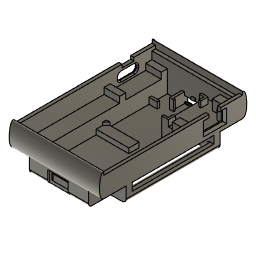
case 9.0 v5 (Autodesk Fusion 360 design; units mm, degrees)
Autodesk Fusion 360 part; units mm, degrees
note: some values were not read from the file. Set by a fixed rule: which face or edge a step refers to.
sketch "case bottom" plane through (0, 0, 0) normal (0, 0, 1) x (1, 0, 0) in component "case"
  line L0 (0, 0) -> (25.8, 0)
  line L1 (25.8, 0) -> (25.8, 34.5)
  line L2 (25.8, 34.5) -> (0, 34.5)
  line L3 (0, 34.5) -> (0, 0)
  line L4 (12.9, 0) -> (12.9, 61.75) construction
  line L5 (8.5, 59.25) -> (17.3, 59.25)
  line L6 (17.3, 59.25) -> (17.3, 64.25)
  line L7 (17.3, 64.25) -> (8.5, 64.25)
  line L8 (8.5, 64.25) -> (8.5, 59.25)
  line L9 (8.5, 59.25) -> (17.3, 64.25) construction
  line L10 (17.3, 59.25) -> (8.5, 64.25) construction
  line L11 (8.35, 64.4) -> (8.35, 59.1)
  line L12 (8.35, 59.1) -> (17.45, 59.1)
  line L13 (17.45, 59.1) -> (17.45, 64.4)
  line L14 (17.45, 64.4) -> (8.35, 64.4)
  line L15 (27.4, 66) -> (-1.6, 66)
  line L16 (-1.6, 66) -> (-1.6, -1.6)
  line L17 (-1.6, -1.6) -> (27.4, -1.6)
  line L18 (27.4, -1.6) -> (27.4, 66)
  line L19 (27.4, 66) -> (-1.6, -1.6) construction
  line L20 (-1.6, 66) -> (27.4, -1.6) construction
  line L21 (-1.6, 32.2) -> (-9.2, 32.2) construction
  line L22 (-9.2, 32.2) -> (-9.2, 12.2)
  line L23 (-5.4, 32.2) -> (-5.4, 12.2)
  line L24 (-5.4, 12.2) -> (-1.6, 12.2)
  line L25 (-1.6, 9.2) -> (-9.2, 9.2)
  line L26 (-9.2, 9.2) -> (-9.2, 12.2)
  line L27 (-5.4, 52.2) -> (-1.6, 52.2)
  line L28 (-5.4, 32.2) -> (-5.4, 52.2)
  line L29 (-1.6, 55.2) -> (-9.2, 55.2)
  line L30 (-9.2, 55.2) -> (-9.2, 52.2)
  line L31 (-9.2, 32.2) -> (-9.2, 52.2)
  line L32 (27.4, 55.2) -> (35, 55.2)
  line L33 (31.2, 52.2) -> (27.4, 52.2)
  line L34 (31.2, 32.2) -> (31.2, 52.2)
  line L35 (35, 55.2) -> (35, 52.2)
  line L36 (35, 32.2) -> (35, 52.2)
  line L37 (31.2, 32.2) -> (31.2, 12.2)
  line L38 (35, 32.2) -> (35, 12.2)
  line L39 (35, 9.2) -> (35, 12.2)
  line L40 (27.4, 9.2) -> (35, 9.2)
  line L41 (31.2, 12.2) -> (27.4, 12.2)
  line L42 (8.35, 64.4) -> (0, 64.4)
  line L43 (0, 64.4) -> (0, 34.5)
  line L44 (17.45, 64.4) -> (25.8, 64.4)
  line L45 (25.8, 64.4) -> (25.8, 34.5)
  line L46 (9.15, 58.3) -> (7.15, 58.3)
  line L47 (7.15, 58.3) -> (7.15, 64.4)
  line L48 (18.65, 58.3) -> (18.65, 64.4)
  line L49 (16.65, 58.3) -> (18.65, 58.3)
  line L50 (25.8, 29.5) -> (0, 29.5)
  line L51 (9.15, 58.3) -> (9.15, 59.1)
  line L52 (16.65, 58.3) -> (16.65, 59.1)
  line L53 (0, 34.5) -> (16, 34.5)
  line L54 (16, 34.5) -> (16, 55.4)
  line L55 (16, 55.4) -> (0, 55.4)
  line L56 (0, 55.4) -> (0, 34.5)
  line L57 (4, 55.4) -> (4, 56.6)
  line L58 (4, 56.6) -> (0, 56.6)
  line L59 (0, 32.7) -> (1.8, 34.5)
  line L60 (0, 32.7) -> (3.5846, 32.7) construction
  line L61 (25.8, 32.7) -> (24, 34.5)
  line L62 (16, 34.5) -> (16, 29.5)
  point P0 (12.9, 43.5)
  point P1 (12.9, 61.75)
  point P2 (12.9, 32.2)
  dimension "d1" = 25.8
  dimension "d2" = 34.5
  dimension "d6" = 8.8
  dimension "d7" = 5
  dimension "d8" = 0.15
  dimension "d10" = 1.6
  dimension "d11" = 1.6
  dimension "d12" = 1.6
  dimension "d13" = 7.6
  dimension "d15" = 3.8
  dimension "d16" = 3
  dimension "d17" = 20
  dimension "d21" = 6.1
  dimension "d23" = 1.2
  dimension "d24" = 5
  dimension "d104" = 29.9
  dimension "d105" = 0.8
  dimension "d106" = 0.8
  dimension "d107" = 16
  dimension "d108" = 20.9
  dimension "d109" = 1.2
  dimension "d110" = 4
  dimension "d155" = 45
  dimension "d156" = 1.8
  constraint horizontal L0
  constraint vertical L1
  constraint horizontal L2
  constraint vertical L3
  constraint coincident L0.start L3.end
  constraint midpoint L0 L4.start
  constraint perpendicular L0 L4
  constraint coincident L4 P0
  constraint horizontal L5
  constraint perpendicular L5 L6
  constraint parallel L5 L7
  constraint parallel L6 L8
  constraint coincident L9 P1
  constraint coincident L10 P1
  constraint coincident P1 L4.end
  constraint horizontal L15
  constraint perpendicular L15 L16
  constraint parallel L15 L17
  constraint parallel L16 L18
  constraint coincident L19 P2
  constraint coincident L20 P2
  constraint coincident L4 P2
  constraint midpoint L16 L21.start
  constraint perpendicular L16 L21
  constraint perpendicular L21 L22
  constraint coincident L21 L23.start
  constraint perpendicular L21 L23
  constraint coincident L16 L24.end
  constraint perpendicular L16 L24
  constraint coincident L16 L25.start
  constraint perpendicular L16 L25
  constraint perpendicular L25 L26
  constraint symmetric L22.start L21 L31.start
  constraint symmetric L21 L22.end L30.end
  constraint symmetric L21 L23.start L28.start
  constraint symmetric L21 L23.end L27.start
  constraint symmetric L21 L24.end L27.end
  constraint symmetric L21 L25.start L29.start
  constraint symmetric L21 L25.end L29.end
  constraint symmetric L4 L21.end L36.start
  constraint symmetric L4 L22.end L38.end
  constraint symmetric L4 L23.start L34.start
  constraint symmetric L4 L23.end L37.end
  constraint symmetric L4 L24.end L41.end
  constraint symmetric L4 L25.start L40.start
  constraint symmetric L4 L25.end L39.start
  constraint symmetric L4 L27.start L33.start
  constraint symmetric L4 L27.end L33.end
  constraint symmetric L4 L29.start L32.start
  constraint symmetric L4 L29.end L32.end
  constraint symmetric L4 L30.end L35.end
  constraint perpendicular L3 L42
  constraint perpendicular L2 L43
  constraint perpendicular L18 L44
  constraint perpendicular L44 L45
  constraint coincident L42 L47.end
  constraint perpendicular L42 L47
  constraint symmetric L4 L46.start L49.start
  constraint symmetric L4 L46.end L48.start
  constraint symmetric L4 L47.end L48.end
  constraint coincident L1 L50.start
  constraint coincident L3 L50.end
  constraint perpendicular L3 L50
  constraint coincident L12 L51.end
  constraint perpendicular L12 L51
  constraint symmetric L4 L51.end L52.end
  constraint horizontal L53
  constraint vertical L54
  constraint horizontal L55
  constraint vertical L56
  constraint coincident L55 L57.start
  constraint perpendicular L55 L57
  constraint coincident L43 L58.end
  constraint perpendicular L43 L58
  constraint horizontal L60
  constraint coincident L3 L59.start
  constraint coincident L53 L59.end
  constraint symmetric L4 L59.start L61.start
  constraint symmetric L4 L59.end L61.end
  constraint coincident L50 L62.end
  constraint perpendicular L50 L62
  measures "d1" distance of L0.start L0.end
  measures "d2" distance of L0.start L2.end
  measures "d6" distance of L6.end L7.end
  measures "d7" distance of L5.start L7.end
  measures "d10" distance of L3 L16
  measures "d11" distance of L0 L17
  measures "d12" distance of L14 L15
  measures "d13" distance of L21.start L21.end
  measures "d15" distance of L16 L23
  measures "d16" distance of L24 L25
  measures "d17" distance of L21 L24
  measures "d21" distance of L46.end L47.end
  measures "d23" distance of L11 L47
  measures "d24" distance of L2 L50
  measures "d104" distance of L2 L42
  measures "d105" distance of L11 L51
  measures "d106" distance of L46.start L51.end
  measures "d107" distance of L2.end L53.end
  measures "d108" distance of L2.end L55.end
  measures "d109" distance of L57.start L57.end
  measures "d110" distance of L57.end L58.end
  measures "d155" angle of L59 L60
  measures "d156" distance of L53 L59.start
extrude "Extrude1" add sketch "case bottom" against normal blind 1.6 contours L0 L1 L3 L50 | L2 L3 L50 L53 L59 L62 | L1 L2 L50 L61 L62 | L2 L3 L53 L59 | L1 L2 L61 | L2 L43 L53 L54 L55 L56 | L2 L12 L42 L43 L44 L45 L46 L47 L48 L49 L51 L52 L54 L55 L57 L58 | L43 L55 L57 L58 | L12 L13 L44 L48 L49 L52 | L11 L12 L13 L14 | L11 L12 L42 L46 L47 L51 | L5 L6 L7 L8 | L15 L16 L17 L18 | L18 L32 L33 L34 L35 L36 L37 L38 L39 L40 L41 | L16 L22 L23 L24 L25 L26 L27 L28 L29 L30 L31 | L18 L33 L34 L37 L41 | L16 L23 L24 L27 L28 makes body 1 in component "case"
extrude "Extrude1'" add sketch "case bottom" along normal blind 3 contours L43 L55 L57 L58 bodies 1 in component "case"
extrude "Extrude2" add sketch "case bottom" along normal blind 5 contours L12 L13 L44 L48 L49 L52 | L11 L12 L42 L46 L47 L51 bodies 1 in component "case"
extrude "Extrude4" add sketch "case bottom" along normal blind 7.6 contours L15 L16 L17 L18 | L18 L32 L33 L34 L35 L36 L37 L38 L39 L40 L41 | L16 L22 L23 L24 L25 L26 L27 L28 L29 L30 L31 | L18 L33 L34 L37 L41 | L16 L23 L24 L27 L28 bodies 1 in component "case"
extrude "Extrude3" add sketch "case bottom" along normal blind 2.4 contours L2 L3 L50 L53 L59 L62 | L2 L3 L53 L59 bodies 1 in component "case"
extrude "Extrude21" add sketch "case bottom" along normal blind 1.4 from surface at 2.4 contours L2 L3 L53 L59 bodies 1 in component "case"
sketch "case top" plane through (0, 0, 7.6) normal (0, 0, 1) x (-1, 0, 0) in component "case"
  line L0 (0, -64.4) -> (-25.8, -64.4)
  line L1 (-25.8, -64.4) -> (-25.8, 0)
  line L2 (-25.8, 0) -> (0, 0)
  line L3 (0, 0) -> (0, -64.4)
  line L4 (1.6, -9.2) -> (1.6, 1.6)
  line L5 (1.6, 1.6) -> (-27.4, 1.6)
  line L6 (-27.4, 1.6) -> (-27.4, -9.2)
  line L7 (-27.4, -9.2) -> (-35, -9.2)
  line L8 (-35, -9.2) -> (-35, -55.2)
  line L9 (-35, -55.2) -> (-27.4, -55.2)
  line L10 (-27.4, -55.2) -> (-27.4, -66)
  line L11 (-27.4, -66) -> (1.6, -66)
  line L12 (1.6, -66) -> (1.6, -55.2)
  line L13 (1.6, -55.2) -> (9.2, -55.2)
  line L14 (9.2, -55.2) -> (9.2, -9.2)
  line L15 (9.2, -9.2) -> (1.6, -9.2)
  line L16 (-12.9, 0) -> (-12.9, -61.75) construction
  line L17 (-25.8, 0) -> (0, 0)
  line L18 (7.6, 0) -> (-33.4, 0)
  line L19 (-33.4, 0) -> (-33.4, -41)
  line L20 (-33.4, -41) -> (7.6, -41)
  line L21 (7.6, -41) -> (7.6, 0)
  line L22 (7.6, 0) -> (-33.4, -41) construction
  line L23 (-33.4, 0) -> (7.6, -41) construction
  line L24 (7.6, -44) -> (-20.9, -44)
  line L25 (-20.9, -44) -> (-20.9, -61.4)
  line L26 (-20.9, -61.4) -> (7.6, -61.4)
  line L27 (7.6, -61.4) -> (7.6, -44)
  line L28 (-20.9, -52.7) -> (7.6, -52.7) construction
  line L29 (-19.2, -47.3) -> (-20.9, -47.3)
  line L30 (-20.9, -47.3) -> (-20.9, -58.1)
  line L31 (-20.9, -58.1) -> (-19.2, -58.1)
  line L32 (-19.2, -58.1) -> (-19.2, -47.3)
  line L33 (-19.2, -47.3) -> (-20.9, -58.1) construction
  line L34 (-20.9, -47.3) -> (-19.2, -58.1) construction
  line L35 (-33.4, -41) -> (-33.4, -64.4)
  line L36 (-31, -41) -> (-31, -64.4)
  line L37 (-33.4, -64.4) -> (7.6, -64.4)
  line L38 (7.6, -64.4) -> (7.6, -41)
  line L39 (-33.4, -52.7) -> (7.6, -52.7) construction
  line L40 (-30.2, -64.4) -> (-30.2, -60.6)
  line L41 (-30.2, -60.6) -> (-24, -60.6)
  line L42 (-24, -60.6) -> (-24, -59.5)
  line L43 (-24, -59.5) -> (-23, -59.5)
  line L44 (-23, -59.5) -> (-23, -57.6)
  line L45 (-23, -57.6) -> (-20, -57.6)
  line L46 (-20, -57.6) -> (-20, -52.7)
  line L47 (-30.2, -41) -> (-30.2, -44.8)
  line L48 (-30.2, -44.8) -> (-24, -44.8)
  line L49 (-24, -44.8) -> (-24, -45.9)
  line L50 (-24, -45.9) -> (-23, -45.9)
  line L51 (-23, -45.9) -> (-23, -47.8)
  line L52 (-23, -47.8) -> (-20, -47.8)
  line L53 (-20, -47.8) -> (-20, -52.7)
  line L54 (9.2, -41) -> (9.2, 1.6)
  line L55 (9.2, 1.6) -> (-35, 1.6)
  line L56 (-35, 1.6) -> (-35, -41)
  line L57 (-35, -41) -> (-35, -66)
  line L58 (-35, -66) -> (9.2, -66)
  line L59 (9.2, -66) -> (9.2, -41)
  line L60 (-31, -52.7) -> (-36, -52.7)
  line L61 (-36, -52.7) -> (-36, -57.7)
  line L62 (-36, -57.7) -> (-31, -57.7)
  line L63 (-36, -52.7) -> (-36, -47.7)
  line L64 (-36, -47.7) -> (-31, -47.7)
  point P0 (-12.9, -20.5)
  point P1 (-20.05, -52.7)
  dimension "d58" = 41
  dimension "d59" = 41
  dimension "d60" = 28.5
  dimension "d61" = 17.4
  dimension "d63" = 1.7
  dimension "d64" = 10.8
  dimension "d66" = 2.4
  dimension "d67" = 23.4
  dimension "d68" = 0.8
  dimension "d69" = 7
  dimension "d70" = 1
  dimension "d71" = 1.1
  dimension "d72" = 4.9
  dimension "d73" = 11
  dimension "d74" = 7.9
  dimension "d75" = 1.6
  dimension "d93" = 5
  dimension "d181" = 0.15
  dimension "d198" = 0.15
  constraint horizontal L18
  constraint perpendicular L18 L19
  constraint parallel L18 L20
  constraint parallel L19 L21
  constraint coincident L22 P0
  constraint coincident L23 P0
  constraint coincident L16 P0
  constraint collinear L2 L18
  constraint horizontal L24
  constraint vertical L25
  constraint horizontal L26
  constraint vertical L27
  constraint collinear L21 L27
  constraint midpoint L25 L28.start
  constraint midpoint L27 L28.end
  constraint horizontal L29
  constraint perpendicular L29 L30
  constraint parallel L29 L31
  constraint parallel L30 L32
  constraint coincident L33 P1
  constraint coincident L34 P1
  constraint coincident L28 P1
  constraint collinear L25 L30
  constraint perpendicular L20 L35
  constraint parallel L35 L36
  constraint coincident L20 L36.start
  constraint perpendicular L27 L37
  constraint perpendicular L20 L38
  constraint midpoint L35 L39.start
  constraint midpoint L38 L28.end
  constraint coincident L36.end L37
  constraint coincident L37 L40.start
  constraint perpendicular L37 L40
  constraint perpendicular L10 L41
  constraint perpendicular L0 L42
  constraint perpendicular L10 L43
  constraint perpendicular L43 L44
  constraint perpendicular L25 L45
  constraint coincident L39 L46.end
  constraint perpendicular L39 L46
  constraint collinear L28 L39
  constraint symmetric L39 L40.start L47.start
  constraint symmetric L39 L40.end L47.end
  constraint symmetric L39 L41.end L48.end
  constraint symmetric L39 L42.end L49.end
  constraint symmetric L39 L43.end L50.end
  constraint symmetric L39 L44.end L51.end
  constraint symmetric L39 L45.end L52.end
  constraint symmetric L39 L46.end L53.end
  constraint midpoint L36 L60.start
  constraint perpendicular L57 L60
  constraint perpendicular L60 L61
  constraint coincident L36 L62.end
  constraint perpendicular L36 L62
  constraint perpendicular L62 L63
  constraint coincident L36 L64.end
  constraint perpendicular L36 L64
  constraint equal L61 L63
  constraint equal L61 L62
  measures "d58" distance of L19.end L20.end
  measures "d59" distance of L18.end L19.end
  measures "d60" distance of L24.start L24.end
  measures "d61" distance of L24.start L26.end
  measures "d63" distance of L30.end L31.end
  measures "d64" distance of L29.end L30.end
  measures "d66" distance of L35 L36
  measures "d67" distance of L19.end L35.end
  measures "d68" distance of L36 L40
  measures "d69" distance of L36 L42
  measures "d70" distance of L42.end L43.end
  measures "d71" distance of L41.end L42.end
  measures "d72" distance of L39 L45
  measures "d73" distance of L36 L46
  measures "d74" distance of L39 L41
  measures "d93" distance of L61.end L62.end
extrude "Extrude5" add sketch "case top" against normal blind 1.6 contours L12 L13 L27 L37 L38 L58 L59 | L12 L26 L37 L38 | L10 L37 L40 L41 | L10 L35 L37 L57 L58 L62 | L12 L13 L26 L27 L38 | L9 L10 L36 L37 L40 L41 | L35 L36 L37 L62 | L9 L35 L36 L62 | L9 L35 L57 L62 | L4 L15 L18 L21 | L4 L15 L18 L21 L54 L55 | L6 L7 L18 L19 L55 L56 | L6 L7 L18 L19 bodies 1 in component "case"
extrude "Extrude6" add sketch "case top" along normal blind 8.4 contours L0 L10 L11 L12 L37 L58 | L12 L13 L27 L37 L38 L58 L59 | L10 L35 L37 L57 L58 L62 | L13 L14 L15 L21 L27 L38 L54 L59 | L2 L4 L5 L6 L17 L18 L55 | L9 L35 L57 L62 | L4 L15 L18 L21 L54 L55 | L6 L7 L18 L19 L55 L56 | L8 L9 L35 L57 L60 | L7 L8 L19 L35 L56 L57 L64 | L8 L35 L57 L60 L64 bodies 1 in component "case"
sketch "case top lift" plane through (0, 0, 0) normal (0, 0, 1) x (-1, 0, 0) in component "case"
  line L0 (-25.8, 0) -> (-25.8, -64.4)
  line L1 (-25.8, -64.4) -> (-18.65, -64.4)
  line L2 (-18.65, -64.4) -> (-18.65, -58.3)
  line L3 (-18.65, -58.3) -> (-16.65, -58.3)
  line L4 (-16.65, -58.3) -> (-16.65, -59.1)
  line L5 (-16.65, -59.1) -> (-17.45, -59.1)
  line L6 (-17.45, -59.1) -> (-17.45, -64.4)
  line L7 (-8.35, -64.4) -> (-8.35, -59.1)
  line L8 (-8.35, -59.1) -> (-9.15, -59.1)
  line L9 (-9.15, -59.1) -> (-9.15, -58.3)
  line L10 (-9.15, -58.3) -> (-7.15, -58.3)
  line L11 (-7.15, -58.3) -> (-7.15, -64.4)
  line L12 (0, -29.5) -> (0, 0)
  line L13 (0, -56.6) -> (-4, -56.6)
  line L14 (-4, -56.6) -> (-4, -55.4)
  line L15 (-4, -55.4) -> (0, -55.4)
  line L16 (0, -34.5) -> (-16, -34.5)
  line L17 (-20.9, -61.4) -> (7.6, -61.4)
  line L18 (-20.9, -44) -> (-20.9, -61.4)
  line L19 (-20.9, -58.1) -> (-19.2, -58.1)
  line L20 (-19.2, -58.1) -> (-19.2, -47.3)
  line L21 (-19.2, -47.3) -> (-20.9, -47.3)
  line L22 (7.6, -44) -> (-20.9, -44)
  line L23 (-30.2, -60.6) -> (-24, -60.6)
  line L24 (-24, -60.6) -> (-24, -59.5)
  line L25 (-24, -59.5) -> (-23, -59.5)
  line L26 (-23, -59.5) -> (-23, -57.6)
  line L27 (-23, -57.6) -> (-20, -57.6)
  line L28 (-20, -57.6) -> (-20, -52.7)
  line L29 (-20, -47.8) -> (-20, -52.7)
  line L30 (-23, -47.8) -> (-20, -47.8)
  line L31 (-23, -45.9) -> (-23, -47.8)
  line L32 (-24, -45.9) -> (-23, -45.9)
  line L33 (-24, -44.8) -> (-24, -45.9)
  line L34 (-30.2, -44.8) -> (-24, -44.8)
  line L35 (-16, -50) -> (-16.65, -50)
  line L36 (-16, -43) -> (-21.9, -43)
  line L37 (-21.9, -43) -> (-21.9, -62.4)
  line L38 (-21.9, -62.4) -> (-18.65, -62.4)
  line L39 (-16.65, -44) -> (-16.65, -43)
  line L40 (-21.9, -43) -> (-25.8, -43)
  line L41 (-16.65, -58.3) -> (-16.65, -59.1)
  line L42 (-16.65, -59.1) -> (-17.45, -59.1)
  line L43 (-17.45, -59.1) -> (-17.45, -64.4)
  line L44 (-17.45, -64.4) -> (-25.8, -64.4)
  line L45 (-17.45, -64.4) -> (-8.35, -64.4)
  line L46 (-7.15, -64.4) -> (0, -64.4)
  line L47 (-20.9, -46.5) -> (-21.9, -46.5)
  line L48 (-18.4, -44) -> (-18.4, -43)
  line L49 (-18.65, -62.4) -> (-17.45, -62.4)
  line L50 (-18.4, -62.4) -> (-18.4, -61.4)
  line L51 (-20.9, -58.9) -> (-21.9, -58.9)
  line L52 (-17.45, -58.3) -> (-17.45, -50)
  line L53 (-16.65, -50) -> (-17.45, -50)
  line L54 (-16, -43) -> (-16, -50)
  line L55 (-17.45, -59.1) -> (-17.45, -58.3)
  line L56 (-16, -34.5) -> (-16, -29.5)
  line L57 (-16, -29.5) -> (0, -29.5)
  line L58 (0, 0) -> (-25.8, 0)
  line L59 (0, -55.4) -> (0, -34.5)
  line L60 (-18.65, -58.3) -> (-18.65, -43)
  line L61 (0, -64.4) -> (0, -56.6)
  dimension "d113" = 1
  dimension "d114" = 1
  dimension "d115" = 1
  dimension "d116" = 7
  dimension "d119" = 2.5
  dimension "d120" = 2.5
  dimension "d121" = 2.5
  dimension "d122" = 2.5
  dimension "d126" = 16
  constraint coincident L22 L39.start
  constraint perpendicular L17 L37
  constraint coincident L2 L38.end
  constraint perpendicular L2 L38
  constraint coincident L36 L39.end
  constraint perpendicular L36 L39
  constraint coincident L0 L40.end
  constraint perpendicular L0 L40
  constraint coincident L3.end L4.start
  constraint coincident L4.end L5.start
  constraint coincident L5.end L6.start
  constraint coincident L6.end L43.end
  constraint coincident L0.end L1.start
  constraint coincident L18 L47.start
  constraint coincident L37 L47.end
  constraint perpendicular L37 L47
  constraint coincident L22 L48.start
  constraint coincident L36 L48.end
  constraint perpendicular L36 L48
  constraint coincident L43 L49.end
  constraint perpendicular L43 L49
  constraint coincident L49 L50.start
  constraint coincident L17 L50.end
  constraint perpendicular L17 L50
  constraint coincident L18 L51.start
  constraint coincident L37 L51.end
  constraint perpendicular L37 L51
  constraint coincident L3 L52.start
  constraint perpendicular L35 L52
  constraint perpendicular L52 L53
  constraint perpendicular L35 L54
  constraint collinear L43 L52
  constraint coincident L2.end L3.start
  constraint coincident L36 L60.end
  constraint perpendicular L36 L60
  measures "d113" distance of L18 L37
  measures "d114" distance of L22 L36
  measures "d115" distance of L17 L38
  measures "d116" distance of L35 L36
  measures "d119" distance of L18 L48
  measures "d120" distance of L22 L47
  measures "d121" distance of L18 L50
  measures "d122" distance of L17 L51
  measures "d126" distance of L12 L54
extrude "Extrude10" add sketch "case top lift" along normal up to surface (7.6 mm away) contours L0 L30 L31 L32 L33 L34 L37 L40 | L0 L23 L24 L25 L26 L27 L30 L31 L32 L33 L34 L37 | L18 L22 L36 L37 L47 L60 | L0 L1 L2 L23 L24 L25 L26 L27 L37 L38 L44 | L18 L30 L37 L47 | L2 L17 L18 L19 L20 L21 L22 L60 | L18 L27 L30 L37 | L18 L27 L28 L29 L30 | L18 L19 L20 L21 L27 L28 L29 L30 | L18 L27 L37 L51 | L2 L17 L18 L37 L38 L51 bodies 1 in component "case"
extrude "Extrude9" add sketch "case top" along normal blind 5 contours L1 L10 L37 L41 | L10 L37 L40 L41 | L1 L20 L47 L48 | L35 L36 L37 L62 | L20 L35 L36 L64 bodies 1 in component "case"
extrude "Extrude11" add sketch "case top lift" along normal blind 3 from surface at 7.6 contours L18 L22 L36 L37 L47 L60 | L2 L17 L18 L37 L38 L51 bodies 1 in component "case"
extrude "Extrude19" add sketch "case top" along normal up to surface (3 mm away) contours L3 L12 L26 L37 | L12 L26 L37 L38 | L3 L20 L24 L38 bodies 1 in component "case"
ref_plane "WorkPlane1" through (31.2, 32.2, 3) normal (0, 1, 0) x (1, 0, 0) in component "case"
sketch "strap hole" plane through (0, 9.2, 0) normal (0, -1, 0) x (1, 0, 0) in component "case"
  line L0 (35, 6) -> (27.4, 6)
  line L1 (27.4, 6) -> (27.4, -1.6)
  line L2 (27.4, -1.6) -> (35, -1.6)
  line L3 (35, -1.6) -> (35, 6)
  line L4 (27.4, -1.6) -> (27.4, 2.2)
  line L5 (31.2, 6) -> (35, 6)
  arc A0 (31.2, 6) -> (27.4, 2.2) centre (31.2, 2.2) ccw
  line L6 (31.2, -1.6) -> (33, -1.6)
  line L7 (35, 0.4) -> (35, 2.2)
  line L8 (35, 2.2) -> (33.2, 2.2)
  line L9 (31.2, 0.2) -> (31.2, -1.6)
  arc A1 (33.2, 2.2) -> (31.2, 0.2) centre (33.2, 0.2) ccw
  dimension "d80" = 3.8
  dimension "d81" = 2
  constraint coincident L1.end L2.start
  constraint coincident L0.start L3.end
  constraint tangent L4 A0
  constraint tangent L5 A0
  constraint horizontal L6
  constraint vertical L7
  constraint horizontal L8
  constraint vertical L9
  constraint midpoint L3 L7.end
  constraint midpoint L2 L6.start
  constraint tangent L9 A1
  constraint tangent L8 A1
  measures "d80" radius of A0
  measures "d81" radius of A1
extrude "Extrude7" cut sketch "strap hole" along normal mid plane 40 from surface at -23 contours L0 L1 L2 L3 L4 L5 A0 L8 L9 A1 bodies 1 in component "case"
ref_plane "WorkPlane2" through (12.9, 32.2, 7.2) normal (1, 0, 0) x (0, -1, 0) in component "case"
mirror "Mirror1" about plane through (12.9, 32.2, 7.2) normal (1, 0, 0) of "Extrude7" in component "case"
fillet "Fillet1" radius 2 2 edges at (35, 32.2, -1.6) (-9.2, 32.2, -1.6) on bodies 1 in component "case"
sketch "switch hole" plane through (35, 0, 0) normal (1, 0, 0) x (0, 1, 0) in component "case"
  line L0 (9.2, 0.4) -> (55.2, 0.4)
  line L1 (55.2, 0.4) -> (55.2, 6)
  line L2 (55.2, 6) -> (66, 6)
  line L3 (66, 6) -> (66, 16)
  line L4 (66, 16) -> (-1.6, 16)
  line L5 (-1.6, 16) -> (-1.6, 6)
  line L6 (-1.6, 6) -> (9.2, 6)
  line L7 (9.2, 6) -> (9.2, 0.4)
  line L8 (52.2, 6) -> (52.2, 2.2)
  line L9 (52.2, 2.2) -> (12.2, 2.2)
  line L10 (12.2, 2.2) -> (12.2, 6)
  line L11 (12.2, 6) -> (52.2, 6)
  line L12 (41, 7.6) -> (66, 7.6)
  line L13 (52.7, 7.6) -> (52.7, 11.2) construction
  line L14 (57.4, 13.6) -> (48, 13.6)
  line L15 (48, 13.6) -> (48, 8.8)
  line L16 (48, 8.8) -> (57.4, 8.8)
  line L17 (57.4, 8.8) -> (57.4, 13.6)
  line L18 (57.4, 13.6) -> (48, 8.8) construction
  line L19 (48, 13.6) -> (57.4, 8.8) construction
  line L20 (49.8, 13.6) -> (49.8, 16)
  line L21 (55.6, 13.6) -> (55.6, 16)
  line L22 (49.8, 14.8) -> (55.6, 14.8) construction
  line L23 (52.7, 14.8) -> (52.7, 11.2) construction
  point P0 (57.7, 7.6)
  point P1 (47.7, 7.6)
  point P2 (52.7, 7.6)
  point P3 (52.7, 11.2)
  dimension "d94" = 9.4
  dimension "d95" = 4.8
  dimension "d96" = 1.2
  dimension "d97" = 5.8
  constraint coincident P2 L13.start
  constraint perpendicular L12 L13
  constraint horizontal L14
  constraint perpendicular L14 L15
  constraint parallel L14 L16
  constraint parallel L15 L17
  constraint coincident L18 P3
  constraint coincident L19 P3
  constraint coincident P3 L13.end
  constraint coincident L14 L20.start
  constraint coincident L4 L20.end
  constraint perpendicular L4 L20
  constraint coincident L14 L21.start
  constraint coincident L4 L21.end
  constraint perpendicular L4 L21
  constraint midpoint L20 L22.start
  constraint midpoint L21 L22.end
  constraint midpoint L22 L23.start
  constraint perpendicular L14 L23
  measures "d94" distance of L15.end L16.end
  measures "d95" distance of L14.end L15.end
  measures "d96" distance of L12 L16
  measures "d97" distance of L20 L21
extrude "Extrude8" cut sketch "switch hole" against normal up to surface (1.6 mm away) contours L4 L14 L20 L21 | L14 L15 L16 L17 bodies 1 in component "case"
sketch "jst hole" plane through (0, 64.4, 0) normal (0, -1, 0) x (1, 0, 0) in component "case"
  line L0 (25.8, 7.6) -> (25.8, 12.6)
  line L1 (25.8, 12.6) -> (30.2, 12.6)
  line L2 (30.2, 12.6) -> (30.2, 7.6)
  line L3 (31, 7.6) -> (31, 12.6)
  line L4 (31, 12.6) -> (33.4, 12.6)
  line L5 (33.4, 12.6) -> (33.4, 16)
  line L6 (33.4, 16) -> (-7.6, 16)
  line L7 (-7.6, 16) -> (-7.6, 10.6)
  line L8 (8.35, 0) -> (17.45, 0)
  line L9 (12.9, 0) -> (12.9, 4.1) construction
  line L10 (17.45, 4.1) -> (8.35, 4.1)
  line L11 (8.35, 4.1) -> (8.35, 0)
  line L12 (8.35, 0) -> (17.45, 0)
  line L13 (17.45, 0) -> (17.45, 4.1)
  line L14 (17.45, 4.1) -> (8.35, 0) construction
  line L15 (8.35, 4.1) -> (17.45, 0) construction
  line L16 (8.35, 0.6) -> (17.45, 0.6)
  line L17 (8.35, 3.5) -> (17.45, 3.5)
  line L18 (13.9, 4.1) -> (11.9, 4.1)
  line L19 (11.9, 4.1) -> (11.9, 4.9)
  line L20 (11.9, 4.9) -> (13.9, 4.9)
  line L21 (13.9, 4.9) -> (13.9, 4.1)
  line L22 (13.9, 4.1) -> (11.9, 4.9) construction
  line L23 (11.9, 4.1) -> (13.9, 4.9) construction
  line L24 (-7.6, 10.6) -> (0, 10.6)
  line L25 (0, 10.6) -> (0, 0)
  line L26 (0, 0) -> (7.15, 0)
  line L27 (7.15, 0) -> (7.15, 5)
  line L28 (7.15, 5) -> (8.35, 5)
  line L29 (8.35, 5) -> (8.35, 0)
  line L30 (8.35, 0) -> (17.45, 0)
  line L31 (17.45, 0) -> (17.45, 5)
  line L32 (18.65, 7.6) -> (25.8, 7.6)
  line L33 (30.2, 7.6) -> (31, 7.6)
  line L34 (18.65, 5) -> (18.65, 7.6)
  line L35 (17.45, 5) -> (18.65, 5)
  point P0 (12.9, 2.05)
  point P1 (12.9, 4.5)
  dimension "d127" = 9.1
  dimension "d128" = 4.1
  dimension "d129" = 0.6
  dimension "d130" = 0.6
  dimension "d131" = 2
  dimension "d132" = 0.8
  constraint midpoint L8 L9.start
  constraint perpendicular L8 L9
  constraint horizontal L10
  constraint perpendicular L10 L11
  constraint parallel L10 L12
  constraint parallel L11 L13
  constraint coincident L14 P0
  constraint coincident L15 P0
  constraint coincident L9 P0
  constraint collinear L8 L12
  constraint coincident L11 L16.start
  constraint horizontal L17
  constraint coincident L11 L17.start
  constraint coincident L13 L17.end
  constraint midpoint L9.end L10
  constraint horizontal L18
  constraint perpendicular L18 L19
  constraint parallel L18 L20
  constraint parallel L19 L21
  constraint coincident L22 P1
  constraint coincident L23 P1
  constraint collinear L9.start L9.end P1
  constraint collinear L10 L18
  measures "d127" distance of L8.start L8.end
  measures "d128" distance of L10.end L8.start
  measures "d129" distance of L10 L17
  measures "d130" distance of L8 L16
  measures "d131" distance of L19.end L20.end
  measures "d132" distance of L18.end L19.end
extrude "Extrude12" cut sketch "jst hole" against normal up to surface (1.6 mm away) contours L11 L13 L16 L17 L29 L31 bodies 1 in component "case"
extrude "Extrude13" cut sketch "jst hole" 1 faces at (14.4167, 64.4, 0.2) along normal up to surface from surface at -0.6 contours L10 L11 L13 L17 L18 L29 L31 end surface through (27.4, 66, 7.6) normal (0, 1, 0) offset 0 on bodies 1 bodies 1 in component "case"
extrude "Extrude14" add sketch "jst hole" along normal blind 0.8 contours L10 L18 L19 L20 L21 bodies 1 in component "case"
chamfer "Chamfer1" distance 0.8 angle 45 1 edges at (12.9, 63.6, 4.9) on bodies 1 in component "case"
sketch "usb-bu hole" plane through (0, 0, 0) normal (0, 1, 0) x (-1, 0, 0) in component "case"
  line L0 (-25.8, 0) -> (0, 0)
  line L1 (0, 0) -> (0, 7.6)
  line L2 (0, 7.6) -> (7.6, 7.6)
  line L3 (7.6, 7.6) -> (7.6, 16)
  line L4 (7.6, 16) -> (-33.4, 16)
  line L5 (-33.4, 16) -> (-33.4, 7.6)
  line L6 (-33.4, 7.6) -> (-25.8, 7.6)
  line L7 (-25.8, 7.6) -> (-25.8, 0)
  line L8 (-25.8, 1.5) -> (-17, 1.5) construction
  line L9 (0, 1.5) -> (-7.8, 1.5) construction
  line L10 (-17, 1.5) -> (-7.8, 1.5) construction
  line L11 (-8.4, 3) -> (-16.4, 3)
  line L12 (-16.4, 3) -> (-16.4, 0)
  line L13 (-16.4, 0) -> (-8.4, 0)
  line L14 (-8.4, 0) -> (-8.4, 3)
  line L15 (-8.4, 3) -> (-16.4, 0) construction
  line L16 (-16.4, 3) -> (-8.4, 0) construction
  line L17 (-7.4, -1.5) -> (-17.4, -1.5)
  line L18 (-17.4, -1.5) -> (-17.4, 4.5)
  line L19 (-17.4, 4.5) -> (-7.4, 4.5)
  line L20 (-7.4, 4.5) -> (-7.4, -1.5)
  line L21 (-7.4, -1.5) -> (-17.4, 4.5) construction
  line L22 (-17.4, -1.5) -> (-7.4, 4.5) construction
  line L23 (-17.4, -1.5) -> (-17.4, -2.5404)
  line L24 (-17.4, -2.5404) -> (-7.4, -2.5404)
  line L25 (-7.4, -2.5404) -> (-7.4, -1.5)
  point P0 (-12.4, 1.5)
  point P1 (-12.4, 1.5)
  dimension "d142" = 8.8
  dimension "d143" = 7.8
  dimension "d145" = 9.2
  dimension "d146" = 8
  dimension "d147" = 3
  dimension "d150" = 10
  dimension "d151" = 6
  constraint coincident L7 L8.start
  constraint perpendicular L7 L8
  constraint coincident L1 L9.start
  constraint perpendicular L1 L9
  constraint parallel L8 L10
  constraint horizontal L11
  constraint perpendicular L11 L12
  constraint parallel L11 L13
  constraint parallel L12 L14
  constraint coincident L15 P1
  constraint coincident L16 P1
  constraint midpoint L10 P1
  constraint collinear L0 L13
  constraint horizontal L17
  constraint perpendicular L17 L18
  constraint parallel L17 L19
  constraint parallel L18 L20
  constraint coincident L21 P1
  constraint coincident L22 P1
  constraint coincident P1 P0
  constraint perpendicular L17 L23
  constraint perpendicular L20 L24
  constraint perpendicular L17 L25
  measures "d142" distance of L8.start L8.end
  measures "d143" distance of L9.start L9.end
  measures "d145" distance of L8.end L9.end
  measures "d146" distance of L12.end L13.end
  measures "d147" distance of L11.end L12.end
  measures "d150" distance of L18.end L19.end
  measures "d151" distance of L17.end L18.end
extrude "Extrude15" cut sketch "usb-bu hole" against normal up to surface (1.6 mm away) contours L0 L11 L12 L13 L14 bodies 1 in component "case"
extrude "Extrude16" cut sketch "usb-bu hole" against normal up to surface (1 mm away) from surface at -0.6 contours L0 L13 L17 L18 L20 | L0 L11 L12 L14 L18 L19 L20 | L17 L23 L24 L25 bodies 1 in component "case"
sketch "usb-c hole" plane through (-7.6, 0, 0) normal (1, 0, 0) x (0, 1, 0) in component "case"
  line L0 (0, 7.6) -> (41, 7.6)
  line L1 (64.4, 10.6) -> (64.4, 16)
  line L2 (64.4, 16) -> (0, 16)
  line L3 (0, 16) -> (0, 7.6)
  line L4 (52.7, 7.6) -> (52.7, 9.2) construction
  line L5 (56, 9.2) -> (49.4, 9.2)
  line L6 (48.1, 10.5) -> (48.1, 11.5)
  line L7 (49.4, 12.8) -> (56, 12.8)
  line L8 (57.3, 11.5) -> (57.3, 10.5)
  line L9 (57.3, 9.2) -> (48.1, 12.8) construction
  line L10 (48.1, 9.2) -> (57.3, 12.8) construction
  arc A0 (49.4, 12.8) -> (48.1, 11.5) centre (49.4, 11.5) ccw
  arc A1 (57.3, 11.5) -> (56, 12.8) centre (56, 11.5) ccw
  arc A2 (56, 9.2) -> (57.3, 10.5) centre (56, 10.5) ccw
  arc A3 (48.1, 10.5) -> (49.4, 9.2) centre (49.4, 10.5) ccw
  line L11 (61.4, 7.6) -> (61.4, 10.6)
  line L12 (41, 10.6) -> (44, 10.6)
  line L13 (41, 7.6) -> (41, 10.6)
  line L14 (44, 10.6) -> (44, 7.6)
  line L15 (44, 7.6) -> (61.4, 7.6)
  line L16 (61.4, 10.6) -> (64.4, 10.6)
  line L17 (49.8, 14.4) -> (55.6, 14.4)
  line L18 (49.8, 16) -> (49.8, 12.8)
  line L19 (55.6, 16) -> (55.6, 12.8)
  point P0 (52.7, 11)
  point P1 (52.7, 14.4)
  dimension "d157" = 1.6
  dimension "d158" = 9.2
  dimension "d159" = 3.6
  dimension "d160" = 1.3
  dimension "d208" = 5.8
  dimension "d209" = 1.6
  constraint perpendicular L0 L4
  constraint horizontal L5
  constraint perpendicular L5 L6
  constraint parallel L5 L7
  constraint parallel L6 L8
  constraint coincident L9 P0
  constraint coincident L10 P0
  constraint coincident L9.end L6
  constraint coincident L9.end L7
  constraint tangent L6 A0
  constraint tangent L7 A0
  constraint coincident L10.end L7
  constraint coincident L10.end L8
  constraint tangent L7 A1
  constraint tangent L8 A1
  constraint equal A0 A1
  constraint coincident L9.start L8
  constraint coincident L9.start L5
  constraint tangent L8 A2
  constraint tangent L5 A2
  constraint equal A0 A2
  constraint coincident L10.start L5
  constraint coincident L10.start L6
  constraint tangent L5 A3
  constraint tangent L6 A3
  constraint equal A0 A3
  constraint coincident L4.end L5
  constraint collinear L4.start L4.end P0
  constraint midpoint L4.start L15
  constraint parallel L2 L17
  constraint coincident L2 L18.start
  constraint coincident L7 L18.end
  constraint perpendicular L7 L18
  constraint coincident L17.start L18
  constraint midpoint L17 P1
  constraint collinear L4.start L4.end P1
  constraint coincident L2 L19.start
  constraint coincident L7 L19.end
  constraint perpendicular L7 L19
  constraint coincident L17.end L19
  measures "d157" distance of L4.start L4.end
  measures "d158" distance of L9.end L10.end
  measures "d159" distance of L10.start L9.end
  measures "d160" radius of A0
  measures "d208" distance of L17.start L17.end
  measures "d209" distance of L2 L17
extrude "Extrude17" cut sketch "usb-c hole" against normal up to surface (1.6 mm away) contours L2 L17 L18 L19 | L5 L6 L7 L8 A0 A1 A2 A3 bodies 1 in component "case"
chamfer "Chamfer2" distance 0.6 angle 45 16 edges at (-7.6, 52.7, 9.2) (-7.6, 48.4808, 9.5808) (-7.6, 48.1, 11) (-7.6, 48.4808, 12.4192) (-7.6, 52.7, 12.8) (-7.6, 56.9192, 12.4192) (-7.6, 57.3, 11) (-7.6, 56.9192, 9.5808) (-9.2, 52.7, 9.2) (-9.2, 56.9192, 9.5808) (-9.2, 57.3, 11) (-9.2, 56.9192, 12.4192) (-9.2, 52.7, 12.8) (-9.2, 48.4808, 12.4192) (-9.2, 48.1, 11) (-9.2, 48.4808, 9.5808) on bodies 1 in component "case"
chamfer "Chamfer3" distance 1 angle 45 5 edges at (35, 56.5, 13.6) (35, 57.4, 11.2) (35, 52.7, 8.8) (35, 48, 11.2) (35, 48.9, 13.6) on bodies 1 in component "case"
fillet "Fillet2" radius 1.6 3 edges at (2.9, -1.6, -1.6) (22.4, -1.6, -1.6) (12.9, 66, -1.6) on bodies 1 in component "case"
fillet "Fillet3" radius 1.6 2 edges at (-1.6, 32.2, -1.6) (27.4, 32.2, -1.6) on bodies 1 in component "case"
sketch "rounded edge" plane through (35, 0, 0) normal (1, 0, 0) x (0, 1, 0) in component "case"
  line L0 (47, 14.6) -> (49.8, 14.6)
  line L1 (49.8, 14.6) -> (49.8, 16)
  line L2 (49.8, 16) -> (-1.6, 16)
  line L3 (-1.6, 16) -> (-1.6, 6)
  line L4 (-1.6, 6) -> (9.2, 6)
  line L5 (9.2, 6) -> (9.2, 0.4)
  line L6 (9.2, 0.4) -> (55.2, 0.4)
  line L7 (55.2, 0.4) -> (55.2, 6)
  line L8 (55.2, 6) -> (66, 6)
  line L9 (66, 6) -> (66, 16)
  line L10 (66, 16) -> (55.6, 16)
  line L11 (55.6, 16) -> (55.6, 14.6)
  line L12 (55.6, 14.6) -> (58.4, 14.6)
  line L13 (58.4, 14.6) -> (58.4, 7.8)
  line L14 (58.4, 7.8) -> (47, 7.8)
  line L15 (47, 7.8) -> (47, 14.6)
  line L16 (52.2, 6) -> (52.2, 2.2)
  line L17 (52.2, 2.2) -> (12.2, 2.2)
  line L18 (12.2, 2.2) -> (12.2, 6)
  line L19 (12.2, 6) -> (52.2, 6)
  line L20 (-1.6, 16) -> (-1.75, 16)
  line L21 (-1.75, 16) -> (-1.75, 17.6)
  line L22 (-1.6, 6) -> (-6.2294, 6) construction
  line L23 (-6.2294, 6) -> (-6.2294, 17.6) construction
  line L24 (-6.2294, 17.6) -> (-1.6, 17.6) construction
  line L25 (-1.6, 17.6) -> (-1.6, 6) construction
  line L26 (-6.2294, 11.8) -> (-1.6, 11.8) construction
  spline S0 degree 5 poles (-1.6, 6) (-2.027, 6) (-2.7708, 6.2369) (-3.5557, 7.3021) (-4.0217, 9.8627) (-3.887, 13.7373) (-3.3197, 16.2979) (-2.6401, 17.3631) (-2.0667, 17.6) (-1.75, 17.6) knots 0 0 0 0 0 0 0.2 0.4 0.6 0.8 1 1 1 1 1 1
  line L27 (-2.2861, 17.6) -> (-1.2139, 17.6)
  line L28 (-0.8709, 6) -> (-2.3291, 6)
  dimension "d169" = 0.15
  dimension "d170" = 1.6
  constraint coincident L2.end L3.start
  constraint perpendicular L3 L20
  constraint perpendicular L20 L21
  constraint horizontal L22
  constraint vertical L23
  constraint horizontal L24
  constraint vertical L25
  constraint coincident L3.end L4.start
  constraint midpoint L23 L26.start
  constraint midpoint L25 L26.end
  constraint midpoint L21.end L27
  constraint coincident L24 L27.start
  constraint parallel L24 L27
  constraint midpoint L3.end L28
  constraint coincident L22 L28.end
  measures "d169" distance of L2.end L20.end
  measures "d170" distance of L20.end L21.end
extrude "Extrude18" add sketch "rounded edge" against normal up to surface (44.2 mm away) contours L3 L20 L21 S0 bodies 1 in component "case"
mirror "Mirror2" about plane through (31.2, 32.2, 3) normal (0, 1, 0) of "Extrude18" in component "case"
sketch "lid, battery section" plane through (0, 0, 16) normal (0, 0, 1) x (-1, 0, 0) in component "case"
  line L0 (-35, -49.8) -> (-33.4, -49.8)
  line L1 (-33.4, -49.8) -> (-33.4, 0)
  line L2 (-33.4, 0) -> (7.6, 0)
  line L3 (7.6, 0) -> (7.6, -49.8)
  line L4 (7.6, -64.4) -> (-33.4, -64.4)
  line L5 (-33.4, -55.6) -> (-35, -55.6)
  line L6 (-35, -55.6) -> (-35, -66.15)
  line L7 (-35, -66.15) -> (9.2, -66.15)
  line L8 (9.2, -49.8) -> (9.2, 1.75)
  line L9 (9.2, 1.75) -> (-35, 1.75)
  line L10 (-35, 1.75) -> (-35, -49.8)
  line L11 (7.6, 0) -> (-33.4, 0)
  line L12 (-33.4, 0) -> (-33.4, 1.75)
  line L13 (7.6, 1.75) -> (7.6, 0)
  line L14 (9.2, 3.2228) -> (-35, 3.2228)
  line L15 (7.6, -49.8) -> (7.6, -66.15)
  line L16 (-33.4, -64.4) -> (-33.4, -66.15)
  line L17 (-35, -67.6228) -> (9.2, -67.6228)
  line L18 (7.6, -49.8) -> (9.2, -49.8)
  line L19 (9.2, -55.6) -> (7.6, -55.6)
  line L20 (7.6, -55.6) -> (7.6, -64.4)
  line L21 (-33.4, -64.4) -> (-33.4, -55.6)
  line L22 (9.2, -66.15) -> (9.2, -55.6)
  constraint horizontal L11
  constraint vertical L12
  constraint vertical L13
  constraint coincident L2.end L3.start
  constraint coincident L9 L13.start
  constraint coincident L9 L12.end
  constraint coincident L1.end L2.start
  constraint coincident L3.end L15.start
  constraint coincident L7 L15.end
  constraint perpendicular L7 L15
  constraint coincident L4.end L16.start
  constraint coincident L7 L16.end
  constraint perpendicular L7 L16
extrude "Extrude20" cut sketch "lid, battery section" against normal blind 1.6 contours L2 L9 L11 L12 L13 | L4 L7 L15 L16 bodies 1 in component "case"
sketch "Sketch1" plane through (0, 0, 0) normal (0, 0, 1) x (1, 0, 0) in component "lid"
  line L0 (-9.2, -1.75) -> (-9.2, 49.8)
  line L1 (-7.6, 55.6) -> (-7.6, 66.15) construction
  line L2 (33.4, 49.8) -> (33.4, -1.75) construction
  line L3 (35, 49.8) -> (33.4, 49.8)
  line L4 (33.4, 55.6) -> (35, 55.6) construction
  line L5 (35, 55.6) -> (35, 66.15)
  line L6 (35, 49.8) -> (35, -1.75)
  line L7 (35, 49.8) -> (35, 55.6)
  line L8 (35, 66) -> (-9.2, 66)
  line L9 (-9.2, -1.6) -> (35, -1.6)
  line L10 (33.25, 49.8) -> (33.25, 0)
  line L11 (-7.45, 64.25) -> (33.25, 64.25)
  line L12 (33.25, 64.25) -> (33.25, 55.6)
  line L13 (-6.65, 0) -> (-6.65, 63.45)
  line L14 (32.45, 63.45) -> (32.45, 55.6)
  line L15 (35, 55.45) -> (32.45, 55.45)
  line L16 (32.45, 55.45) -> (32.45, 55.6)
  line L17 (33.25, 55.6) -> (33.25, 55.45)
  line L18 (33.4, -1.75) -> (-7.6, -1.75) construction
  line L19 (-7.6, 0) -> (33.4, 0)
  line L20 (-7.45, 0) -> (-7.45, -1.6)
  line L21 (33.25, 0) -> (33.25, -1.6)
  line L22 (31, 41) -> (33.4, 41)
  line L23 (35, 49.95) -> (32.45, 49.95)
  line L24 (32.45, 55.45) -> (32.45, 49.95)
  line L25 (32.45, 49.95) -> (32.45, 0)
  line L26 (32.45, 63.45) -> (32.45, 64.25)
  line L27 (-6.65, 63.45) -> (-6.65, 64.25)
  line L28 (33.25, 64.25) -> (33.25, 66)
  line L29 (33.25, 49.8) -> (33.25, 49.95)
  line L30 (-7.45, 64.25) -> (-7.45, 66)
  line L31 (-7.6, -1.75) -> (-9.2, -1.75) construction
  line L32 (-7.6, 66.15) -> (-9.2, 66.15) construction
  line L33 (-9.2, 55.6) -> (-9.2, 66.15)
  line L34 (-7.6, -1.75) -> (-7.6, 49.8) construction
  line L35 (33.4, 49.8) -> (33.4, -1.75) construction
  line L36 (33.4, 66.15) -> (33.4, 55.6) construction
  line L37 (35, -1.75) -> (33.4, -1.75) construction
  line L38 (35, 66.15) -> (33.4, 66.15) construction
  line L39 (0, 41) -> (-7.6, 41)
  line L40 (12.9, 64.25) -> (12.9, 0) construction
  line L41 (-9.2, 55.45) -> (-6.65, 55.45)
  line L42 (-9.2, 49.8) -> (-9.2, 55.6)
  line L43 (-9.2, 49.95) -> (-6.65, 49.95)
  line L44 (-7.45, 0) -> (-7.45, 49.95)
  line L45 (-7.45, 55.45) -> (-7.45, 64.25)
  dimension "d193" = 0.15
  dimension "d194" = 0.8
  dimension "d197" = 0.15
  dimension "d199" = 0.15
  dimension "d200" = 0.15
  dimension "d206" = 0.15
  dimension "d207" = 0.8
  dimension "d210" = 0.15
  constraint coincident L3.start L6.start
  constraint coincident L4.end L5.start
  constraint coincident L5 L8.start
  constraint coincident L0 L8.end
  constraint perpendicular L0 L8
  constraint coincident L0 L9.start
  constraint coincident L6 L9.end
  constraint perpendicular L6 L9
  constraint coincident L7 L15.start
  constraint perpendicular L7 L15
  constraint perpendicular L15 L16
  constraint coincident L15 L17.end
  constraint perpendicular L15 L17
  constraint parallel L2 L10
  constraint parallel L1 L44
  constraint parallel L1 L13
  constraint collinear L10 L12
  constraint coincident L20.start L19
  constraint coincident L13.start L19
  constraint coincident L10.end L19
  constraint coincident L9 L20.end
  constraint perpendicular L9 L20
  constraint coincident L9 L21.end
  constraint perpendicular L9 L21
  constraint coincident L7 L23.start
  constraint perpendicular L16 L23
  constraint perpendicular L23 L24
  constraint coincident L19 L25.end
  constraint perpendicular L19 L25
  constraint coincident L11 L26.end
  constraint perpendicular L11 L26
  constraint coincident L11 L27.end
  constraint perpendicular L11 L27
  constraint coincident L8 L28.end
  constraint perpendicular L8 L28
  constraint coincident L23 L29.end
  constraint perpendicular L23 L29
  constraint coincident L8 L30.end
  constraint perpendicular L8 L30
  constraint midpoint L11 L40.start
  constraint midpoint L19 L40.end
  constraint perpendicular L19 L40
  constraint symmetric L3.start L40 L0.end
  constraint symmetric L4.end L40 L33.start
  constraint symmetric L15.start L40 L41.start
  constraint symmetric L15.end L40 L41.end
  constraint symmetric L23.start L40 L43.start
  constraint symmetric L23.end L40 L43.end
  constraint coincident L43 L44.end
  constraint coincident L41 L45.start
  constraint collinear L14 L26
  constraint perpendicular L41 L45
  measures "d193" distance of L9 L18
  measures "d194" distance of L13 L44
  measures "d197" distance of L1 L44
  measures "d199" distance of L2 L10
  measures "d200" distance of L4 L15
  measures "d206" distance of L3 L23
  measures "d207" distance of L10 L25
  measures "d210" distance of L8 L32
extrude "Extrude1''" add sketch "Sketch1" along normal blind 1.6 separate body makes body 2 in component "lid"
extrude "Extrude2'" add sketch "Sketch1" against normal blind 1.6 contours L9 L19 L20 L21 | L13 L41 L42 L43 | L13 L39 L43 L44 | L11 L13 L27 L41 L45 | L10 L22 L23 L25 L29 | L8 L11 L28 L30 | L7 L15 L23 L24 | L11 L12 L14 L15 L16 L17 L26 bodies 2 in component "lid"
chamfer "Chamfer1'" distance 0.2 angle 45 1 edges at (35, 52.7, -1.6) on bodies 2 in component "lid"
component "case" placed x (1, 0, 0) y (0, 1, 0) z (0, 0, 1) at (0, 0, 0)
component "lid" placed x (1, 0, 0) y (0, 1, 0) z (0, 0, 1) at (0, 0, 16)
equation "d121 = d119"
equation "d122 = d120"
equation "d197 = d193"
equation "d198 = d197"
equation "d199 = d198"
equation "d200 = d181"
equation "d206 = d200"
equation "d207 = d194"
